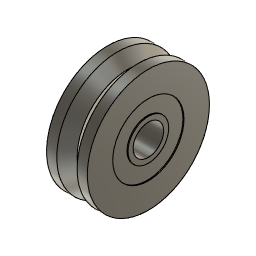
Omni_wheel_r18_FIN v1 (Autodesk Fusion 360 archive; units mm, degrees)
design "rollers"
Autodesk Fusion 360 part; units mm, degrees
sketch "Sketch2" plane through (0, 0, 0) normal (0, 0, 1) x (1, 0, 0)
  line L0 (0, 0) -> (0, 6)
  line L1 (4, 6) -> (4, 0)
  line L2 (4, 0) -> (0, 0)
  line L3 (1, 6) -> (2, 5)
  line L4 (2, 5) -> (3, 6)
  line L5 (0, 6) -> (1, 6)
  line L6 (3, 6) -> (4, 6)
  dimension "d12" = 4
  dimension "d13" = 1
  dimension "d14" = 1
  dimension "d15" = 6
  constraint coincident L0.start L2.end
  constraint coincident L4.end L5
  constraint perpendicular L3 L4
  constraint perpendicular L0 L2
  constraint vertical L0
  constraint horizontal L6
  measures "d12" distance of L0 L1
  measures "d13" distance of L0.end L3.start
  measures "d14" distance of L1.start L4.end
  measures "d15" distance of L2 L5
revolve "Revolve1" add sketch "Sketch2" angle 360 about axis through (4, 0, 0) along (-1, 0, 0)
sketch "Sketch3" plane through (4, 0, 0) normal (1, 0, 0) x (0, 1, 0)
  circle A0 centre (0, 0) radius 6
  circle A1 centre (0, 0) radius 1.5
  dimension "d18" = 3
  constraint coincident A0.centre A1.centre
  measures "d18" diameter of A1
extrude "Extrude2" cut sketch "Sketch3" against normal through all contours A1
sketch "Sketch4" plane through (4, 0, 0) normal (1, 0, 0) x (0, 1, 0)
  circle A0 centre (0, 0) radius 1.5
  circle A1 centre (0, 0) radius 6
  circle A2 centre (0, 0) radius 3.5
  circle A3 centre (0, 0) radius 2
  dimension "d20" = 7
  dimension "d21" = 4
  constraint coincident A0.centre A1.centre
  constraint concentric A2 A3
  measures "d20" diameter of A2
  measures "d21" diameter of A3
extrude "Extrude3" cut sketch "Sketch4" against normal blind 0.1 contours A2
sketch "Sketch5" plane through (0, 0, 0) normal (-1, 0, 0) x (0, -1, 0)
  circle A0 centre (0, 0) radius 1.5
  circle A1 centre (0, 0) radius 6
  circle A2 centre (0, 0) radius 2
  circle A3 centre (0, 0) radius 3.5
  dimension "d24" = 7
  dimension "d25" = 4
  constraint coincident A0.centre A1.centre
  measures "d24" diameter of A3
  measures "d25" diameter of A2
extrude "Extrude4" cut sketch "Sketch5" against normal blind 0.1 contours A3

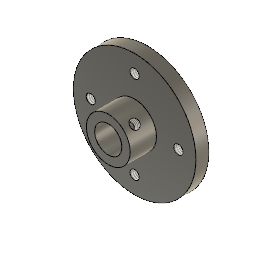
design "Omni_wheel_disk"
Autodesk Fusion 360 part; units mm, degrees
sketch "Sketch1" plane through (0, 0, 0) normal (0, 1, 0) x (1, 0, 0)
  circle A0 centre (0, 0) radius 14
  circle A1 centre (0, -10) radius 1.25
  line L0 (0, 0) -> (0, -14) construction
  circle A2 centre (10, 0) radius 1.25
  circle A3 centre (0, 10) radius 1.25
  circle A4 centre (-10, 0) radius 1.25
  dimension "d1" = 28
  dimension "d7" = 2.5
  dimension "d8" = 10
  dimension "d10" = 360
  constraint coincident A0.centre L0.start
  constraint coincident A0 L0.end
  constraint vertical L0
  constraint coincident A1.centre L0
  measures "d1" diameter of A0
  measures "d7" diameter of A1
  measures "d8" distance of A0.centre A1.centre
extrude "Extrude1" add sketch "Sketch1" along normal blind 3
sketch "Sketch2" plane through (0, 0, 0) normal (0, -1, 0) x (1, 0, 0)
  circle A0 centre (0, 0) radius 14
  circle A1 centre (0, 0) radius 5
  circle A2 centre (-10, 0) radius 1.25
  circle A3 centre (0, 10) radius 1.25
  circle A4 centre (0, -10) radius 1.25
  circle A5 centre (10, 0) radius 1.25
  dimension "d4" = 10
  constraint coincident A0.centre A1.centre
  measures "d4" diameter of A1
extrude "Extrude2" add sketch "Sketch2" along normal blind 6 contours A1
thread "Thread1" "ISO Metric profile 2.5 M2.5x0.45 6H" major diameter 2.58 minor diameter 2.0755 pitch 0.45 angle 60 resizes the face on face at (11.2484, 2, 0.0623) on face at (1.2484, 2, -9.9377) on face at (-8.7516, 2, 0.0623) on face at (1.2484, 2, 10.0623)
sketch "Sketch3" plane through (0, -6, 0) normal (0, -1, 0) x (1, 0, 0)
  circle A0 centre (0, 0) radius 5
  circle A1 centre (0, 0) radius 3.1
  dimension "d11" = 6.2
  constraint concentric A0 A1
  measures "d11" diameter of A1
extrude "Extrude3" cut sketch "Sketch3" against normal through all contours A1
sketch "Sketch5" plane through (0, 0, 0) normal (0, 0, 1) x (1, 0, 0)
  circle A0 centre (0, -3.5) radius 1.25
  line L0 (-5, -6) -> (5, -6)
  dimension "d13" = 2.5
  dimension "d14" = 2.5
  dimension "d15" = 5
  measures "d13" diameter of A0
  measures "d14" distance of A0.centre L0
  measures "d15" horizontal distance of A0.centre L0.end
extrude "Extrude4" cut sketch "Sketch5" along normal through all
move_face "MoveFace1" to x (0.707107, 0, -0.707107) y (0, 1, 0) z (0.707107, 0, 0.707107) at (0, 0, 0) 1 faces at (0.6905, -2.458, 4.3076)
thread "Thread2" "ISO Metric profile 2.5 M2.5x0.45 6H" major diameter 2.58 minor diameter 2.0755 pitch 0.45 angle 60 resizes the face on face at (3.7523, -2.8756, 2.2209)
